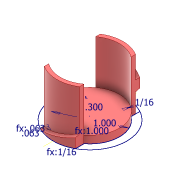
# Autodesk Inventor part: Chalk Holder
Saved by Autodesk Inventor 2020.4 (Build 244396000, 396)
## iProperties
Created: 2022-05-28
Part Number: Chalk Holder
Material: Generic
Document SubType Name: Modeling
Designer: david
Density: 1 g/cm^3
Appearance: Smooth - Red
Author: david
Autodesk Inventor part; units mm, degrees
ref_plane "YZ Plane" through (0, 0, 0) normal (1, 0, 0) x (0, 1, 0)
ref_plane "XZ Plane" through (0, 0, 0) normal (0, 1, 0) x (-1, 0, 0)
ref_plane "XY Plane" through (0, 0, 0) normal (0, 0, 1) x (1, 0, 0)
sketch "Sketch1" plane through (0, 0, 0) normal (0, 1, 0) x (-1, 0, 0)
  circle A0 centre (0, 0) radius 12.7
  line L0 (7.62, -12.0859) -> (7.62, 12.0859)
  line L1 (0, -6.2891) -> (0, 4.9731)
  line L2 (-7.62, -12.0859) -> (-7.62, 12.0859)
  arc A1 (7.62, 12.0859) -> (-7.62, 12.0859) centre (0, 0) ccw
  arc A2 (-7.62, -12.0859) -> (7.62, -12.0859) centre (0, 0) ccw
  point P0 (7.62, -10.16)
  point P1 (-7.62, -10.16)
  point P2 (-7.62, 10.16)
  point P3 (7.62, 10.16)
  dimension "d0" = 25.4
  dimension "d10" = 1.5875
  dimension "d11" = 1.5875
  dimension "d12" = 7.62
  constraints: 6 end point, 4 point on circle, 3 centre point, 2 coincident, 2 symmetric about line, 2 vertical
  measures "d0" diameter of A0
  measures "d10" radial gap between concentric circles of A2 A0
  measures "d11" radial gap between concentric circles of A1 A0
  measures "d12" distance between parallel lines of L1 L0
extrude "Extrusion3" add sketch "Sketch1" along normal blind 22.225 contours A0 L2 A1 L0 | L0 A2 L2 A0
extrude "Extrusion4" add sketch "Sketch1" along normal blind 3.175 contours A0 L0 | L0 A0 L2 | L2 A0
sketch "Sketch2" plane through (0, 0, 0) normal (0, -1, 0) x (1, 0, 0)
  arc A0 (7.62, 12.0859) -> (-7.62, 12.0859) centre (0, 0) ccw projected
  line L0 (7.62, 12.0859) -> (7.62, 10.16) projected
  line L1 (7.62, 12.0859) -> (7.62, 13.9266)
  line L2 (-7.62, 12.0859) -> (-7.62, 13.9266)
  arc A1 (7.62, 13.9266) -> (-7.62, 13.9266) centre (0, 0) ccw
  arc A2 (7.62, 13.9266) -> (-7.62, 13.9266) centre (0, 0) ccw
  circle A3 centre (0, 0) radius 15.875
  circle A4 centre (0, 0) radius 12.7
  line L3 (-7.62, 10.16) -> (-7.62, 12.0859) projected
  line L4 (-7.62, 13.9266) -> (-7.62, 10.16)
  arc A5 (-7.62, -10.16) -> (7.62, -10.16) centre (0, 0) ccw projected
  line L5 (7.62, -10.16) -> (7.62, -13.9266)
  line L6 (7.62, -10.16) -> (7.62, -12.0859) projected
  line L7 (-7.62, -12.0859) -> (-7.62, -10.16) projected
  line L8 (-7.62, -10.16) -> (-7.62, -13.9266)
  point P0 (-7.62, 13.9266)
  dimension "d22" = 1.5875
  dimension "d23" = 1.5875
  dimension "d24" = 25.4
  constraints: 10 end point, 6 point on circle, 4 centre point, 4 collinear, 3 coincident, 1 parallel
  measures "d22" radial gap between concentric circles of A1 A0
  measures "d23" radial gap between concentric circles of A3 A0
  measures "d24" diameter of A4
coil "Coil1" sketch "Sketch2" operation add axis through (0, -10, 0) along (0, 1, 0) pitch 25.4 turns 0.75 hand right contours A0 L2 A1 L1
extrude "Extrusion5" cut sketch "Sketch2" against normal blind 25.4 contours L1 A3 L5 A4 L0 | L3 A4 L7 L8 A3 L2
equation "\"d11\" = d10"
equation "\"d23\" = d22"
equation "\"d24\" = d0"
body "Solid2"
